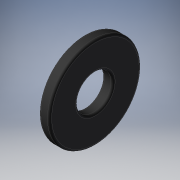
# Autodesk Inventor part: 51200 Shaft washer
Saved by Autodesk Inventor 2019 (Build 230136000, 136)
## iProperties
Created: 2023-01-10
Part Number: 51200 Shaft washer
Material: Generic
Catalog Web Link: www.cadenas.de
Description: With flat seet SW-
Vendor: NSK_RB
Document SubType Name: Modeling
Designer: psAdmin
Manufacturer: NSK_RB
Mass: 1.33383 g
Surface Area: 11.9793 cm^2
Volume: 1.33383 cm^3
Density: 1 g/cm^3
Appearance: PSOLRGB-175-175-175
Category: PARTsolutions
Company: NSK_RB
Title: 51200 Shaft washer
Author: Cadenas PARTsolutions
PSOL_IDENT_0: {$CADENAS_DATA/23d-libs/nsk_rb/roller_bearings/thrust_bearings/single_direction_tbb/with_flat_seet_s
PSOL_IDENT_1: w.prj},189 {VTYP=3D},{NB=51200 Shaft washer},{LINA=51200 Shaft washer},{NN=With flat seet SW},{DATE=
PSOL_IDENT_2: 27.09.2022 23:23:10},{GEOMDATE=23.08.2022 10:45:55},{VERSION=},{LINEID=6260},{WBVAR=},{WBNUMERIC=}
PSOL_IDENT_3: {NB=51200 Shaft washer},{LINA=51200 Shaft washer},{KT=DUMMY},{IDNR=},{STAN=},{NO=2},{ORDER=51200},{S
PSOL_IDENT_4: D=10},{D=26},{T=11},{T3=11.6},{T4=13},{SR=0.6},{CAN=12800},{COAN=17100},{CA=1300},{COA=1740},{GRE=60
PSOL_IDENT_5: 00},{OIL=9000},{SD1=26},{D1=12},{D2=18},{D3=28},{SB=3.5},{A=8.5},{R=22},{SDA=20},{DA=16},{SRA=0.6},{
PSOL_IDENT_6: MASS=0.028},{N=10},{DIST=1.233}
NB: 51200 Shaft washer
NN: With flat seet SW
NBSYN: $ORDER. Shaft washer
LINA: 51200 Shaft washer
CATALOG: NSK Rolling Bearing
NO: 2
ORDER: 51200
SD: 10
D: 26
T: 11
T3: 11.6
T4: 13
SR: 0.6
CAN: 12800
COAN: 17100
CA: 1300
COA: 1740
GRE: 6000
OIL: 9000
SD1: 26
D1: 12
D2: 18
D3: 28
SB: 3.5
A: 8.5
R: 22
SDA: 20
DA: 16
SRA: 0.6
MASS: 0.028
N: 10
SUPPLIER: NSK_RB
ARTICLENO: 51200 Shaft washer
BOMINFO: 51200 Shaft washer
CREATOR: CADENAS GmbH
Autodesk Inventor part; units mm, degrees
sketch "Sketch_1" plane through (0, 0, 0) normal (0, 0, 1) x (1, 0, 0)
  line L0 (3.0556, 0) -> (0, 0)
  arc A0 (0, 8.2402) -> (0, 10.7598) centre (-2.4444, 9.5) ccw
  line L1 (0, 8.2402) -> (0, 5.6)
  arc A1 (0, 5.6) -> (0.6, 5) centre (0.6, 5.6) ccw
  line L2 (0.6, 5) -> (2.4556, 5)
  arc A2 (2.4556, 5) -> (3.0556, 5.6) centre (2.4556, 5.6) ccw
  line L3 (3.0556, 5.6) -> (3.0556, 12.4)
  arc A3 (3.0556, 12.4) -> (2.4556, 13) centre (2.4556, 12.4) ccw
  line L4 (2.4556, 13) -> (0.6, 13)
  arc A4 (0.6, 13) -> (0, 12.4) centre (0.6, 12.4) ccw
  line L5 (0, 12.4) -> (0, 10.7598)
  constraints: 12 end point, 10 point on circle, 5 centre point
revolve "Revolution1" add sketch "Sketch_1" angle 360 about axis through (3.0556, 0, 0) along (1, 0, 0)
ref_plane "SW_HW_XY" through (-7.9444, 0, 0) normal (1, 0, 0) x (0, 0, -1)
ref_plane "SW_HW_YZ" through (-7.9444, 0, 0) normal (0, 0, -1) x (0, 1, 0)
ref_plane "SW_HW_ZX" through (-7.9444, 0, 0) normal (0, 1, 0) x (1, 0, 0)
body "Solid1"
